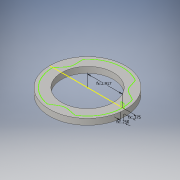
# Autodesk Inventor part: vexCamRing9
Saved by Autodesk Inventor 2016 SP1 (Build 200210100, 210)
## iProperties
Created: 2015-11-02
Part Number: vexCamRing9
Material: Generic
Document SubType Name: Modeling
Designer: steele
Density: 1 g/cm^3
Appearance: Default
Author: steele
Autodesk Inventor part; units mm, degrees
ref_plane "YZ Plane" through (0, 0, 0) normal (1, 0, 0) x (0, 1, 0)
ref_plane "XZ Plane" through (0, 0, 0) normal (0, 1, 0) x (-1, 0, 0)
ref_plane "XY Plane" through (0, 0, 0) normal (0, 0, 1) x (1, 0, 0)
sketch "Sketch1" plane through (0, 0, 0) normal (0, 1, 0) x (-1, 0, 0)
  circle A0 centre (0, 0) radius 55.0333
  circle A1 centre (0, 0) radius 80.4333
  dimension "d0" = 110.0667
  dimension "d1" = 160.8667
  constraints: 2 centre point, 2 coincident
  measures "d0" diameter of A0
  measures "d1" diameter of A1
extrude "Extrusion1" add sketch "Sketch1" against normal blind 12.7
sketch "Sketch2" plane through (0, 0, 0) normal (0, 1, 0) x (1, 0, 0)
  point P0 (0, 0)
  point P1 (69.6156, 25.338)
  point P2 (37.0417, 64.158)
  point P3 (-56.7511, 47.6198)
  point P4 (-56.7511, 47.6198)
  point P5 (-74.0833, 0)
  point P6 (-12.8644, -72.9578)
  point P7 (37.0417, -64.158)
  constraints: 18 other
sketch "Sketch4" plane through (0, 0, 0) normal (0, 0, 1) x (1, 0, 0)
  line L0 (70.9083, -9.525) -> (77.2583, -9.525)
  line L1 (77.2583, -9.525) -> (77.2583, 9.525)
  line L2 (77.2583, 9.525) -> (70.9083, 9.525)
  line L3 (70.9083, 9.525) -> (70.9083, -9.525)
  line L4 (-80.4333, 0) -> (80.4333, 0) projected
  line L5 (70.9083, -9.525) -> (77.2583, 9.525) construction
  line L6 (77.2583, -9.525) -> (70.9083, 9.525) construction
  point P0 (0, 0)
  point P1 (74.0833, 0)
  dimension "d19" = 74.0833
  dimension "d20" = 9.525
  dimension "d21" = 6.35
  constraints: 12 end point, 2 midpoint, 2 parallel, 1 perpendicular, 1 point on line
  measures "d19" distance of point (0, 0) point (74.083, 0)
  measures "d20" distance from line of L0 point (74.083, 0)
  measures "d21" distance of L0.start L0.end
equation "\"d0\" = ringInnerDiam"
equation "\"d1\" = ringOuterDiam"
equation "\"d2\" = ringThickness"
equation "\"ringOuterDiam\" = ringInnerDiam + 2 * ringWidth"
equation "\"ringInnerDiam\" = 110.06667"
equation "\"ringWidth\" = 25.4"
equation "\"ringInnerRadius\" = 0.5 * ringInnerDiam"
equation "\"ringOuterRadius\" = 0.5 * ringOuterDiam"
equation "\"ringThickness\" = 12.7"
equation "\"camOuterRadius\" = -0.5 * camTrackWidth + ringOuterRadius - camTrackSpacing"
equation "\"camTrackWidth\" = 6.35"
equation "\"camTrackSpacing\" = 3.175"
equation "\"camInnerRadius\" = 0.5 * camTrackWidth + ringInnerRadius + camTrackSpacing"
equation "\"camRun\" = camOuterRadius - camInnerRadius"
equation "\"angleScaleFactor\" = 4.5"
equation "\"angle280Delta\" = 1170"
equation "\"camTrackDepth\" = 9.525"
body "Solid1"
